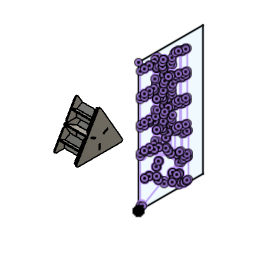
Table and Chair v10 (Autodesk Fusion 360 design; units mm, degrees)
Autodesk Fusion 360 part; units mm, degrees
note: some values were not read from the file. Chosen so that the rebuilt part matches the saved one: which bodies a step acts on.
(part 1 of 4)
sketch "Sketch1" plane through (0, 0, 0) normal (1, 0, 0) x (0, 1, 0)
  line L0 (0, 527.9291) -> (-457.2, -263.9645)
  line L1 (-457.2, -263.9645) -> (457.2, -263.9645)
  line L2 (457.2, -263.9645) -> (0, 527.9291)
  line L3 (0, 0) -> (0, 527.9291) construction
  line L4 (0, 0) -> (-228.6, 131.9823) construction
  line L5 (0, 0) -> (0, -263.9645) construction
  line L6 (0, 0) -> (228.6, 131.9823) construction
  line L7 (-228.6, 131.9823) -> (228.6, 131.9823)
  line L8 (-228.6, 131.9823) -> (0, -263.9645)
  line L9 (0, -263.9645) -> (228.6, 131.9823)
  line L10 (-114.3, -65.9911) -> (-228.6, -131.9823) construction
  line L11 (-228.6, -131.9823) -> (-342.9, -65.9911) construction
  line L12 (-228.6, -131.9823) -> (-228.6, -263.9645) construction
  line L13 (-118.8, -58.1969) -> (-228.6, -121.59)
  line L14 (-228.6, -121.59) -> (-338.4, -58.1969)
  line L15 (-109.8, -73.7854) -> (-219.6, -137.1784)
  line L16 (-219.6, -137.1784) -> (-219.6, -263.9645)
  line L17 (-237.6, -137.1784) -> (-347.4, -73.7854)
  line L18 (-237.6, -137.1784) -> (-237.6, -263.9645)
  line L19 (-228.6, -121.59) -> (-237.6, -137.1784)
  line L20 (-228.6, -121.59) -> (-219.6, -137.1784)
  line L21 (-219.6, -137.1784) -> (-237.6, -137.1784)
  line L22 (-228.6, 113.9823) -> (-441.6115, -254.9645)
  line L23 (-441.6115, -254.9645) -> (-15.5885, -254.9645)
  line L24 (-15.5885, -254.9645) -> (-228.6, 113.9823)
  line L25 (0, 10.3923) -> (-224.1, 139.7765)
  line L26 (0, 10.3923) -> (224.1, 139.7765)
  line L27 (-9, -5.1962) -> (-233.1, 124.188)
  line L28 (-9, -5.1962) -> (-9, -263.9645)
  line L29 (9, -5.1962) -> (9, -263.9645)
  line L30 (9, -5.1962) -> (233.1, 124.188)
  line L31 (-9, -5.1962) -> (9, -5.1962)
  line L32 (0, 10.3923) -> (9, -5.1962)
  line L33 (-9, -5.1962) -> (0, 10.3923)
  line L34 (0, 0, 0) -> (0, 0, 60) construction
  line L35 (-228.6, -131.9823, 0) -> (-228.6, -131.9823, 60) construction
  dimension "d693" = 3.05
  constraint coincident L3.start L4.start
  constraint equal L0 L1
  constraint equal L1 L2
  constraint vertical L3
  constraint midpoint L0 L4.end
  constraint midpoint L1 L5.end
  constraint midpoint L2 L6.end
  constraint equal L4 L6
  constraint equal L4 L5
  constraint midpoint L8 L10.start
  constraint perpendicular L8 L10
  constraint coincident L0 L11.end
  constraint coincident L1 L12.end
  constraint perpendicular L1 L12
  constraint perpendicular L0 L11
  constraint equal L10 L11
  constraint perpendicular L16 L23
  constraint parallel L8 L24
  constraint parallel L0 L22
  measures "d1" distance of L0.start L0.end
  measures "d6" distance of L0 L22
  measures "d7" distance of L1 L23
  measures "d8" distance of L8 L24
  measures "d35" distance of L3.start L4.start
  measures "d36" distance of L10.end L11.start
extrude "Extrude1" add sketch "Sketch1" along normal blind 18 makes body 1
extrude "Extrude2" add sketch "Sketch1" against normal blind 410 separate body contours L8 L9 L28 L29 L31 | L1 L9 L29 | L1 L8 L28 makes body 2
pattern_circular "C-Pattern1" count 3 over 360 about axis through (0, 0, 0) along (1, 0, 0) of bodies 2 makes body 3 at (-136.6667, 79.2, 35.3338) makes body 4 at (-273.3333, -70.2, 50.9223)
extrude "Extrude3" add sketch "Sketch1" against normal blind 18 from surface at -18 separate body contours L13 L14 L22 L24 | L14 L17 L19 L22 | L13 L15 L20 L24 | L17 L18 L22 L23 | L19 L20 L21 | L15 L16 L23 L24 | L16 L18 L21 L23 makes body 5
sketch "Sketch2" plane through (-410, 0, 0) normal (-1, 0, 0) x (0, -1, 0)
  line L0 (-224.1, 139.7765) -> (-233.1, 124.188)
  line L1 (-233.1, 124.188) -> (-9, -5.1962)
  line L2 (-9, -5.1962) -> (0, 10.3923)
  line L3 (0, 10.3923) -> (-224.1, 139.7765)
  line L4 (233.1, 124.188) -> (224.1, 139.7765)
  line L5 (224.1, 139.7765) -> (0, 10.3923)
  line L6 (0, 10.3923) -> (9, -5.1962)
  line L7 (9, -5.1962) -> (233.1, 124.188)
  line L8 (-9, -263.9645) -> (9, -263.9645)
  line L9 (9, -263.9645) -> (9, -5.1962)
  line L10 (9, -5.1962) -> (-9, -5.1962)
  line L11 (-9, -5.1962) -> (-9, -263.9645)
  line L12 (9, -134.5803) -> (-9, -134.5803) construction
  line L13 (9, -179.5803) -> (-9, -179.5803)
  line L14 (9, -89.5803) -> (-9, -89.5803)
  line L15 (-224.1, 139.7765) -> (224.1, 139.7765)
  line L16 (-233.1, 124.188) -> (-9, -263.9645)
  line L17 (233.1, 124.188) -> (9, -263.9645)
  line L18 (-4.5, 2.5981) -> (9, -5.1962) construction
  line L19 (0, -5.1962) -> (0, 10.3923) construction
  line L20 (73.0789, 52.5844) -> (82.0789, 36.9959)
  line L21 (151.0211, 97.5844) -> (160.0211, 81.9959)
  line L22 (-82.0789, 36.9959) -> (-73.0789, 52.5844)
  line L23 (-160.0211, 81.9959) -> (-151.0211, 97.5844)
  dimension "d34" = 90
  dimension "d38" = 360
  constraint midpoint L9 L12.start
  constraint midpoint L11 L12.end
  constraint coincident L9 L13.start
  constraint coincident L11 L13.end
  constraint perpendicular L11 L13
  constraint coincident L9 L14.start
  constraint coincident L11 L14.end
  constraint perpendicular L11 L14
  constraint symmetric L12 L13 L14
  constraint coincident L0.start L3.end
  constraint coincident L4.end L5.start
  constraint coincident L0.end L1.start
  constraint coincident L8.start L11.end
  constraint coincident L7 L4.start
  constraint coincident L8.end L9.start
  constraint coincident L4.start L7.end
  constraint midpoint L2 L18.start
  constraint coincident L6.end L7.start
  constraint midpoint L10 L19.start
  constraint coincident L2.end L3.start
  constraint coincident L19 origin
  constraint coincident L18 origin
  measures "d34" distance of L13 L14
extrude "Extrude5" add sketch "Sketch2" along normal blind 18 separate body contours L0 L1 L3 L23 | L3 L5 L15 | L1 L11 L16 | L4 L5 L7 L21 | L8 L9 L11 L13 | L1 L2 L3 L22 | L7 L9 L17 | L2 L6 L10 | L5 L6 L7 L20 | L9 L10 L11 L14 makes body 6
extrude "Extrude6" add sketch "Sketch2" along normal blind 18 contours L1 L3 L22 L23 | L5 L7 L20 L21 | L9 L11 L13 L14 bodies 2 3 4
ref_plane "WorkPlane2" through (-205, 0, -134.5803) normal (-1, 0, 0) x (0, 0, 1)
mirror "Mirror2" about plane through (-205, 0, -134.5803) normal (-1, 0, 0) of "Extrude6"
combine "Combine1" operation cut target body 1 tool bodies 3 2 4 keep tools
move_face "OffsetFaces1" offset -0.1 24 faces at (6, -3, -179.5803) (6, -3, -89.5803) (12, 99.0596, 67.5844) (12, 9, -119.5803) (12, -99.0596, 67.5844) (6, 108.0596, 51.9959) (6, -9, -119.5803) (12, -108.0596, 51.9959) (6, 157.0211, 87.1921) (6, -76.0789, 47.3883) (6, 79.0789, 42.1921) (6, -154.0211, 92.3883) (-416, 79.0789, 42.1921) (-416, 157.0211, 87.1921) (-416, 99.0596, 67.5844) (-422, 134.0404, 66.9959) (-416, -76.0789, 47.3883) (-416, -154.0211, 92.3883) (-416, 9, -119.5803) (-416, -125.0404, 82.5844) (-416, -3, -89.5803) (-416, -108.0596, 51.9959) (-416, -3, -179.5803) (-416, -9, -149.5803) on bodies 1 6
ref_plane "WorkPlane1" through (-223, 0, -62.094) normal (-1, 0, 0) x (0, 0, 1)
fillet "Fillet1" radius 30 6 edges at (9, -457.2, -263.9645) (9, 457.2, -263.9645) (9, 0, 527.9291) (-27, -441.6115, -254.9645) (-27, -15.5885, -254.9645) (-27, -228.6, 113.9823) on bodies 1 5
mirror "Mirror1" about plane through (-223, 0, -62.094) normal (-1, 0, 0) of bodies 5 makes body 7
extrude "Extrude4" add sketch "Sketch1" against normal up to surface (374 mm away) from surface at -36 separate body contours L16 L18 L21 L23 makes body 8
pattern_circular "C-Pattern2" count 3 over 360 about axis through (0, -228.6, -131.9823) along (1, 0, 0) of bodies 8 makes body 9 at (-285.3333, -185.5981, -117.5474) makes body 10 at (-160.6667, -262.6019, -101.9589)
sketch "Sketch3" plane through (-428, 0, 0) normal (-1, 0, 0) x (0, -1, 0)
  arc A0 (254.5808, 68.9823) -> (202.6192, 68.9823) centre (228.6, 53.9823) ccw
  line L0 (202.6192, 68.9823) -> (41.5692, -209.9645)
  arc A1 (41.5692, -209.9645) -> (67.55, -254.9645) centre (67.55, -224.9645) ccw
  line L1 (67.55, -254.9645) -> (389.65, -254.9645)
  arc A2 (389.65, -254.9645) -> (415.6308, -209.9645) centre (389.65, -224.9645) ccw
  line L2 (415.6308, -209.9645) -> (254.5808, 68.9823)
  line L3 (339.6058, -78.2854) -> (330.6058, -62.6969)
  line L4 (330.6058, -62.6969) -> (228.6, -121.59)
  line L5 (228.6, -121.59) -> (237.6, -137.1784)
  line L6 (237.6, -137.1784) -> (339.6058, -78.2854)
  line L7 (126.5942, -62.6969) -> (117.5942, -78.2854)
  line L8 (117.5942, -78.2854) -> (219.6, -137.1784)
  line L9 (219.6, -137.1784) -> (228.6, -121.59)
  line L10 (228.6, -121.59) -> (126.5942, -62.6969)
  line L11 (219.6, -254.9645) -> (237.6, -254.9645)
  line L12 (237.6, -254.9645) -> (237.6, -137.1784)
  line L13 (237.6, -137.1784) -> (219.6, -137.1784)
  line L14 (219.6, -137.1784) -> (219.6, -254.9645)
  line L15 (168.5971, -107.7319) -> (177.5971, -92.1434) construction
  line L16 (146.9465, -95.2319) -> (155.9465, -79.6434)
  line L17 (190.2477, -120.2319) -> (199.2477, -104.6434)
  line L18 (228.6, -121.59) -> (228.6, -137.1784)
  line L19 (224.1, -129.3842) -> (237.6, -137.1784)
  line L20 (237.6, -221.0715) -> (219.6, -221.0715)
  line L21 (237.6, -171.0715) -> (219.6, -171.0715)
  line L22 (301.2535, -79.6434) -> (310.2535, -95.2319)
  line L23 (257.9523, -104.6434) -> (266.9523, -120.2319)
  point P0 (228.6, -131.9823)
  dimension "d45" = 50
  dimension "d47" = 360
  constraint midpoint L8 L15.start
  constraint midpoint L10 L15.end
  constraint coincident L8 L16.start
  constraint coincident L10 L16.end
  constraint perpendicular L10 L16
  constraint coincident L8 L17.start
  constraint coincident L10 L17.end
  constraint perpendicular L10 L17
  constraint symmetric L15 L16 L17
  constraint coincident L4.end L5.start
  constraint midpoint L13 L18.end
  constraint midpoint L9 L19.start
  constraint coincident L5.end L6.start
  constraint coincident L19 P0
  constraint coincident L18 P0
  measures "d45" distance of L16 L17
extrude "Extrude7" add sketch "Sketch3" against normal up to surface (18 mm away) separate body contours L4 L6 L22 L23 | L8 L10 L16 L17 | L12 L14 L20 L21 makes body 11 at (-422, -281.386, -111.8986) makes body 12 at (-428, -181.814, -101.5063) makes body 13 at (-422, -219.6, -187.7382)
ref_plane "WorkPlane3" through (-223, -228.6, -70.4911) normal (-1, 0, 0) x (0, 0, 1)
mirror "Mirror3" about plane through (-223, -228.6, -70.4911) normal (-1, 0, 0) of bodies 13 12 11 makes body 14 at (-24, -281.386, -111.8986) makes body 15 at (-18, -181.814, -101.5063) makes body 16 at (-24, -219.6, -187.7382)
combine "Combine2" operation add target body 9 tool bodies 12 15
combine "Combine3" operation add target body 10 tool bodies 11 14
combine "Combine4" operation add target body 8 tool bodies 13 16
combine "Combine5" operation cut target body 5 tool bodies 8 9 10 keep tools
combine "Combine6" operation cut target body 7 tool bodies 10 8 9 keep tools
move_face "OffsetFaces2" offset -0.1 24 faces at (-416, -237.6, -187.7382) (-422, -175.814, -111.8986) (-416, -219.6, -187.7382) (-422, -286.8198, -87.9768) (-422, -193.2477, -115.0357) (-422, -231.6, -171.0715) (-422, -231.6, -221.0715) (-416, -281.386, -111.8986) (-422, -304.2535, -84.8396) (-422, -184.814, -96.3101) (-422, -260.9523, -109.8396) (-422, -149.9465, -90.0357) (-24, -231.6, -171.0715) (-24, -304.2535, -84.8396) (-24, -281.386, -111.8986) (-30, -184.814, -96.3101) (-24, -231.6, -221.0715) (-30, -219.6, -187.7382) (-24, -193.2477, -115.0357) (-30, -272.386, -96.3101) (-30, -237.6, -187.7382) (-30, -175.814, -111.8986) (-24, -260.9523, -109.8396) (-24, -149.9465, -90.0357) on bodies 5 7
pattern_circular "C-Pattern3" count 3 over 360 about axis through (661.68, 0.1832, -0.2415) along (-1, 0, 0) of bodies 7 5 8 9 10 makes body 17 at (-18, -77.6648, 228.6417) makes body 18 at (-18, 237.326, -47.2647) makes body 19 at (-428, -77.6648, 228.6417) makes body 20 at (-428, 237.326, -47.2647) makes body 21 at (-285.3333, -43.302, 299.4332) makes body 22 at (-160.6667, 281.4517, -112.4195) makes body 23 at (-285.3333, -8.516, 208.0051) makes body 24 at (-285.3333, 184.8797, -96.831) makes body 25 at (-285.3333, 67.7038, 292.178) makes body 26 at (-285.3333, 219.6657, -204.9258)
copy_body "Body->Comp1" bodies 1 removing the originals makes body 27 in component "Component"
copy_body "Body->Comp2" bodies 2 removing the originals makes body 28 in component "Component'"
copy_body "Body->Comp3" bodies 3 removing the originals makes body 29 in component "Component''"
copy_body "Body->Comp4" bodies 4 removing the originals makes body 30 in component "Component'''"
copy_body "Body->Comp5" bodies 5 removing the originals makes body 31 in component "Component''''"
copy_body "Body->Comp6" bodies 6 removing the originals makes body 32 in component "Component'''''"
copy_body "Body->Comp7" bodies 7 removing the originals makes body 33 in component "Component''''''"
copy_body "Body->Comp8" bodies 8 removing the originals makes body 34 in component "Component'''''''"
copy_body "Body->Comp9" bodies 9 removing the originals makes body 35 in component "Component''''''''"
copy_body "Body->Comp10" bodies 10 removing the originals makes body 36 in component "Component'''''''''"
copy_body "Body->Comp11" bodies 17 removing the originals makes body 37 in component "Component''''''''''"
copy_body "Body->Comp12" bodies 18 removing the originals makes body 38 in component "Component'''''''''''"
copy_body "Body->Comp13" bodies 19 removing the originals makes body 39 in component "Component''''''''''''"
copy_body "Body->Comp14" bodies 20 removing the originals makes body 40 in component "Component'''''''''''''"
copy_body "Body->Comp15" bodies 21 removing the originals makes body 41 in component "Component''''''''''''''"
copy_body "Body->Comp16" bodies 22 removing the originals makes body 42 in component "Component'''''''''''''''"
copy_body "Body->Comp17" bodies 23 removing the originals makes body 43 in component "Component''''''''''''''''"
copy_body "Body->Comp18" bodies 24 removing the originals makes body 44 in component "Component'''''''''''''''''"
copy_body "Body->Comp19" bodies 25 removing the originals makes body 45 in component "Component''''''''''''''''''"
copy_body "Body->Comp20" bodies 26 removing the originals makes body 46 in component "Component'''''''''''''''''''"
sketch "Sketch4" plane through (18, 0, 0) normal (1, 0, 0) x (0, 1, 0)
  arc A0 (25.9808, 482.9291) -> (-25.9808, 482.9291) centre (0, 467.9291) ccw
  line L0 (-25.9808, 482.9291) -> (-431.2192, -218.9645)
  arc A1 (-431.2192, -218.9645) -> (-405.2385, -263.9645) centre (-405.2385, -233.9645) ccw
  line L1 (-405.2385, -263.9645) -> (405.2385, -263.9645)
  arc A2 (405.2385, -263.9645) -> (431.2192, -218.9645) centre (405.2385, -233.9645) ccw
  line L2 (431.2192, -218.9645) -> (25.9808, 482.9291)
  line L3 (-72.9423, 52.621) -> (-82.0423, 36.8593)
  line L4 (-82.0423, 36.8593) -> (-160.1577, 81.9593)
  line L5 (-160.1577, 81.9593) -> (-151.0577, 97.721)
  line L6 (-151.0577, 97.721) -> (-72.9423, 52.621)
  line L7 (-9.1, -89.4803) -> (9.1, -89.4803)
  line L8 (9.1, -89.4803) -> (9.1, -179.6803)
  line L9 (9.1, -179.6803) -> (-9.1, -179.6803)
  line L10 (-9.1, -179.6803) -> (-9.1, -89.4803)
  line L11 (82.0423, 36.8593) -> (72.9423, 52.621)
  line L12 (72.9423, 52.621) -> (151.0577, 97.721)
  line L13 (151.0577, 97.721) -> (160.1577, 81.9593)
  line L14 (160.1577, 81.9593) -> (82.0423, 36.8593)
  line L15 (700, 919.2) -> (3138.4, 919.2)
  line L16 (3138.4, 919.2) -> (3138.4, -1519.2)
  line L17 (3138.4, -1519.2) -> (700, -1519.2)
  line L18 (700, -1519.2) -> (700, 919.2)
  dimension "d53" = 2438.4
  dimension "d54" = 2438.4
  constraint horizontal L15
  constraint vertical L16
  constraint horizontal L17
  constraint vertical L18
  measures "d53" distance of L15.start L15.end
  measures "d54" distance of L15.start L17.end
extrude "Extrude1'" add sketch "Sketch4" along normal blind 1 separate body contours L15 L16 L17 L18 makes body 47 in component "sheet"
other "Arrange1"
ref_plane "WorkPlane56" through (39, 1561.7871, -1471.2) normal (1, 0, 0) x (0, 0, 1)
sketch "Sketch58" plane through (39, 1561.7871, -1471.2) normal (1, 0, 0) x (0, 0, 1)
  line L0 (0, 0) -> (0, 33.8931) construction
  line L1 (-18, 0) -> (0, 0) construction
  line L2 (0, 0) -> (-2.1567, 2.1567) construction
  circle A0 centre (-2.1567, 2.1567) radius 3.05
  dimension "d525" = 3.05
  constraint coincident L0.start L1.end
  constraint coincident L0.start A0
  measures "d525" distance of L0.start L2.end
sweep "Sweep5" cut profiles "Sketch58" along 1 edges at (-410, -151.4465, -87.4377) section 1 sketch seen with x (0, -0.5, 0.866025) y (0, -0.866025, -0.5) z (1, 0, 0) at (1061.2, 1225.1008, 651.8867) on bodies 35 bodies 35 in component "Component''''''''"
ref_plane "WorkPlane57" through (57, 1611.7871, -1471.2) normal (-1, 0, 0) x (0, 0, -1)
sketch "Sketch59" plane through (57, 1611.7871, -1471.2) normal (-1, 0, 0) x (0, 0, -1)
  line L0 (0, 0) -> (0, -33.8931) construction
  line L1 (18, 0) -> (0, 0) construction
  line L2 (0, 0) -> (2.1567, -2.1567) construction
  circle A0 centre (2.1567, -2.1567) radius 3.05
  dimension "d533" = 3.05
  constraint coincident L0.start L1.end
  constraint coincident L0.start A0
  measures "d533" distance of L0.start L2.end
sweep "Sweep6" cut profiles "Sketch59" along 1 edges at (-410, -194.7477, -112.4377) section 1 sketch seen with x (0, -0.5, 0.866025) y (0, -0.866025, -0.5) z (1, 0, 0) at (1061.2, 1225.1008, 651.8867) on bodies 35 bodies 35 in component "Component''''''''"
ref_plane "WorkPlane58" through (57, 1561.7871, -1097.2) normal (-1, 0, 0) x (0, 0, -1)
sketch "Sketch60" plane through (57, 1561.7871, -1097.2) normal (-1, 0, 0) x (0, 0, -1)
  line L0 (0, 0) -> (0, 33.8931) construction
  line L1 (-18, 0) -> (0, 0) construction
  line L2 (0, 0) -> (-2.1567, 2.1567) construction
  circle A0 centre (-2.1567, 2.1567) radius 3.05
  dimension "d541" = 3.05
  constraint coincident L0.start L1.end
  constraint coincident L0.start A0
  measures "d541" distance of L0.start L2.end
sweep "Sweep7" cut profiles "Sketch60" along 1 edges at (-36, -151.4465, -87.4377) section 1 sketch seen with x (0, -0.5, 0.866025) y (0, -0.866025, -0.5) z (1, 0, 0) at (1061.2, 1225.1008, 651.8867) on bodies 35 bodies 35 in component "Component''''''''"
ref_plane "WorkPlane59" through (39, 1611.7871, -1097.2) normal (1, 0, 0) x (0, 0, 1)
sketch "Sketch61" plane through (39, 1611.7871, -1097.2) normal (1, 0, 0) x (0, 0, 1)
  line L0 (0, 0) -> (0, -33.8931) construction
  line L1 (18, 0) -> (0, 0) construction
  line L2 (0, 0) -> (2.1567, -2.1567) construction
  circle A0 centre (2.1567, -2.1567) radius 3.05
  dimension "d549" = 3.05
  constraint coincident L0.start L1.end
  constraint coincident L0.start A0
  measures "d549" distance of L0.start L2.end
sweep "Sweep8" cut profiles "Sketch61" along 1 edges at (-36, -194.7477, -112.4377) section 1 sketch seen with x (0, -0.5, 0.866025) y (0, -0.866025, -0.5) z (1, 0, 0) at (1061.2, 1225.1008, 651.8867) on bodies 35 bodies 35 in component "Component''''''''"
ref_plane "WorkPlane60" through (57, 1611.7872, -1041.2) normal (-1, 0, 0) x (0, 0, -1)
sketch "Sketch62" plane through (57, 1611.7872, -1041.2) normal (-1, 0, 0) x (0, 0, -1)
  line L0 (0, 0) -> (0, -33.8931) construction
  line L1 (18, 0) -> (0, 0) construction
  line L2 (0, 0) -> (2.1567, -2.1567) construction
  circle A0 centre (2.1567, -2.1567) radius 3.05
  dimension "d557" = 3.05
  constraint coincident L0.start L1.end
  constraint coincident L0.start A0
  measures "d557" distance of L0.start L2.end
sweep "Sweep5'" cut profiles "Sketch62" along 1 edges at (-36, -262.4523, -112.4377) section 1 sketch seen with x (0, 0.5, 0.866025) y (0, 0.866025, -0.5) z (-1, 0, 0) at (-1077.2, -1682.3009, 651.8867) on bodies 36 bodies 36 in component "Component'''''''''"
ref_plane "WorkPlane61" through (39, 1561.7872, -1041.2) normal (1, 0, 0) x (0, 0, 1)
sketch "Sketch63" plane through (39, 1561.7872, -1041.2) normal (1, 0, 0) x (0, 0, 1)
  line L0 (0, 0) -> (0, 33.8931) construction
  line L1 (-18, 0) -> (0, 0) construction
  line L2 (0, 0) -> (-2.1567, 2.1567) construction
  circle A0 centre (-2.1567, 2.1567) radius 3.05
  dimension "d565" = 3.05
  constraint coincident L0.start L1.end
  constraint coincident L0.start A0
  measures "d565" distance of L0.start L2.end
sweep "Sweep6'" cut profiles "Sketch63" along 1 edges at (-36, -305.7535, -87.4377) section 1 sketch seen with x (0, 0.5, 0.866025) y (0, 0.866025, -0.5) z (-1, 0, 0) at (-1077.2, -1682.3009, 651.8867) on bodies 36 bodies 36 in component "Component'''''''''"
ref_plane "WorkPlane62" through (39, 1424.0012, -937.046) normal (1, 0, 0) x (0, 0, 1)
sketch "Sketch64" plane through (39, 1424.0012, -937.046) normal (1, 0, 0) x (0, 0, 1)
  line L0 (0, 0) -> (0, 33.8931) construction
  line L1 (-18, 0) -> (0, 0) construction
  line L2 (0, 0) -> (-2.1567, 2.1567) construction
  circle A0 centre (-2.1567, 2.1567) radius 3.05
  dimension "d573" = 3.05
  constraint coincident L0.start L1.end
  constraint coincident L0.start A0
  measures "d573" distance of L0.start L2.end
sweep "Sweep5''" cut profiles "Sketch64" along 1 edges at (-410, 305.8192, -87.9586) section 1 sketch seen with x (0, -0.5, 0.866025) y (0, -0.866025, -0.5) z (1, 0, 0) at (527.046, 1563.0405, 582.4728) on bodies 42 bodies 42 in component "Component'''''''''''''''"
ref_plane "WorkPlane63" through (57, 1474.0012, -937.046) normal (-1, 0, 0) x (0, 0, -1)
sketch "Sketch65" plane through (57, 1474.0012, -937.046) normal (-1, 0, 0) x (0, 0, -1)
  line L0 (0, 0) -> (0, -33.8931) construction
  line L1 (18, 0) -> (0, 0) construction
  line L2 (0, 0) -> (2.1567, -2.1567) construction
  circle A0 centre (2.1567, -2.1567) radius 3.05
  dimension "d581" = 3.05
  constraint coincident L0.start L1.end
  constraint coincident L0.start A0
  measures "d581" distance of L0.start L2.end
sweep "Sweep6''" cut profiles "Sketch65" along 1 edges at (-410, 262.518, -112.9586) section 1 sketch seen with x (0, -0.5, 0.866025) y (0, -0.866025, -0.5) z (1, 0, 0) at (527.046, 1563.0405, 582.4728) on bodies 42 bodies 42 in component "Component'''''''''''''''"
ref_plane "WorkPlane64" through (57, 1561.7872, -667.2) normal (-1, 0, 0) x (0, 0, -1)
sketch "Sketch66" plane through (57, 1561.7872, -667.2) normal (-1, 0, 0) x (0, 0, -1)
  line L0 (0, 0) -> (0, 33.8931) construction
  line L1 (-18, 0) -> (0, 0) construction
  line L2 (0, 0) -> (-2.1567, 2.1567) construction
  circle A0 centre (-2.1567, 2.1567) radius 3.05
  dimension "d589" = 3.05
  constraint coincident L0.start L1.end
  constraint coincident L0.start A0
  measures "d589" distance of L0.start L2.end
sweep "Sweep7'" cut profiles "Sketch66" along 1 edges at (-410, -305.7535, -87.4377) section 1 sketch seen with x (0, 0.5, 0.866025) y (0, 0.866025, -0.5) z (-1, 0, 0) at (-1077.2, -1682.3009, 651.8867) on bodies 36 bodies 36 in component "Component'''''''''"
ref_plane "WorkPlane65" through (39, 1611.7872, -667.2) normal (1, 0, 0) x (0, 0, 1)
sketch "Sketch67" plane through (39, 1611.7872, -667.2) normal (1, 0, 0) x (0, 0, 1)
  line L0 (0, 0) -> (0, -33.8931) construction
  line L1 (18, 0) -> (0, 0) construction
  line L2 (0, 0) -> (2.1567, -2.1567) construction
  circle A0 centre (2.1567, -2.1567) radius 3.05
  dimension "d597" = 3.05
  constraint coincident L0.start L1.end
  constraint coincident L0.start A0
  measures "d597" distance of L0.start L2.end
sweep "Sweep8'" cut profiles "Sketch67" along 1 edges at (-410, -262.4523, -112.4377) section 1 sketch seen with x (0, 0.5, 0.866025) y (0, 0.866025, -0.5) z (-1, 0, 0) at (-1077.2, -1682.3009, 651.8867) on bodies 36 bodies 36 in component "Component'''''''''"
ref_plane "WorkPlane66" through (39, 1474.0012, -563.046) normal (1, 0, 0) x (0, 0, 1)
sketch "Sketch68" plane through (39, 1474.0012, -563.046) normal (1, 0, 0) x (0, 0, 1)
  line L0 (0, 0) -> (0, -33.8931) construction
  line L1 (18, 0) -> (0, 0) construction
  line L2 (0, 0) -> (2.1567, -2.1567) construction
  circle A0 centre (2.1567, -2.1567) radius 3.05
  dimension "d605" = 3.05
  constraint coincident L0.start L1.end
  constraint coincident L0.start A0
  measures "d605" distance of L0.start L2.end
sweep "Sweep7''" cut profiles "Sketch68" along 1 edges at (-36, 262.518, -112.9586) section 1 sketch seen with x (0, -0.5, 0.866025) y (0, -0.866025, -0.5) z (1, 0, 0) at (527.046, 1563.0405, 582.4728) on bodies 42 bodies 42 in component "Component'''''''''''''''"
ref_plane "WorkPlane67" through (57, 1424.0012, -563.046) normal (-1, 0, 0) x (0, 0, -1)
sketch "Sketch69" plane through (57, 1424.0012, -563.046) normal (-1, 0, 0) x (0, 0, -1)
  line L0 (0, 0) -> (0, 33.8931) construction
  line L1 (-18, 0) -> (0, 0) construction
  line L2 (0, 0) -> (-2.1567, 2.1567) construction
  circle A0 centre (-2.1567, 2.1567) radius 3.05
  dimension "d613" = 3.05
  constraint coincident L0.start L1.end
  constraint coincident L0.start A0
  measures "d613" distance of L0.start L2.end
sweep "Sweep8''" cut profiles "Sketch69" along 1 edges at (-36, 305.8192, -87.9586) section 1 sketch seen with x (0, -0.5, 0.866025) y (0, -0.866025, -0.5) z (1, 0, 0) at (527.046, 1563.0405, 582.4728) on bodies 42 bodies 42 in component "Component'''''''''''''''"
ref_plane "WorkPlane68" through (57, 1589.3944, -543.0459) normal (-1, 0, 0) x (0, 0, -1)
sketch "Sketch70" plane through (57, 1589.3944, -543.0459) normal (-1, 0, 0) x (0, 0, -1)
  line L0 (0, 0) -> (0, -33.8931) construction
  line L1 (18, 0) -> (0, 0) construction
  line L2 (0, 0) -> (2.1567, -2.1567) construction
  circle A0 centre (2.1567, -2.1567) radius 3.05
  dimension "d621" = 3.05
  constraint coincident L0.start L1.end
  constraint coincident L0.start A0
  measures "d621" distance of L0.start L2.end
sweep "Sweep5'''" cut profiles "Sketch70" along 1 edges at (-36, -33.3682, 283.3056) section 1 sketch seen with x (0, 0.5, 0.866025) y (0, 0.866025, -0.5) z (-1, 0, 0) at (-579.0459, -1433.8242, 1036.4336) on bodies 41 bodies 41 in component "Component''''''''''''''"
ref_plane "WorkPlane69" through (39, 1539.3944, -543.0459) normal (1, 0, 0) x (0, 0, 1)
sketch "Sketch71" plane through (39, 1539.3944, -543.0459) normal (1, 0, 0) x (0, 0, 1)
  line L0 (0, 0) -> (0, 33.8931) construction
  line L1 (-18, 0) -> (0, 0) construction
  line L2 (0, 0) -> (-2.1567, 2.1567) construction
  circle A0 centre (-2.1567, 2.1567) radius 3.05
  dimension "d629" = 3.05
  constraint coincident L0.start L1.end
  constraint coincident L0.start A0
  measures "d629" distance of L0.start L2.end
sweep "Sweep6'''" cut profiles "Sketch71" along 1 edges at (-36, -76.6695, 308.3056) section 1 sketch seen with x (0, 0.5, 0.866025) y (0, 0.866025, -0.5) z (-1, 0, 0) at (-579.0459, -1433.8242, 1036.4336) on bodies 41 bodies 41 in component "Component''''''''''''''"
ref_plane "WorkPlane70" through (39, 1401.6083, -507.0458) normal (1, 0, 0) x (0, 0, 1)
sketch "Sketch72" plane through (39, 1401.6083, -507.0458) normal (1, 0, 0) x (0, 0, 1)
  line L0 (-18, 0) -> (0, 0) construction
  line L1 (0, 33.8931) -> (0, 0) construction
  line L2 (0, 0) -> (-2.1567, 2.1567) construction
  circle A0 centre (-2.1567, 2.1567) radius 3.05
  dimension "d637" = 3.05
  constraint coincident L0.end L1.end
  constraint coincident L0.end A0
  measures "d637" distance of L0.end L2.end
sweep "Sweep5''''" cut profiles "Sketch72" along 1 edges at (-36, 151.5122, -87.9586) section 1 sketch seen with x (0, 0.5, 0.866025) y (0, 0.866025, -0.5) z (-1, 0, 0) at (-543.0458, -1086.3162, 571.2763) on bodies 44 bodies 44 in component "Component'''''''''''''''''"
ref_plane "WorkPlane71" through (57, 1451.6083, -507.0458) normal (-1, 0, 0) x (0, 0, -1)
sketch "Sketch73" plane through (57, 1451.6083, -507.0458) normal (-1, 0, 0) x (0, 0, -1)
  line L0 (0, 0) -> (0, -33.8931) construction
  line L1 (18, 0) -> (0, 0) construction
  line L2 (0, 0) -> (2.1567, -2.1567) construction
  circle A0 centre (2.1567, -2.1567) radius 3.05
  dimension "d645" = 3.05
  constraint coincident L0.start L1.end
  constraint coincident L0.start A0
  measures "d645" distance of L0.start L2.end
sweep "Sweep6''''" cut profiles "Sketch73" along 1 edges at (-36, 194.8135, -112.9586) section 1 sketch seen with x (0, 0.5, 0.866025) y (0, 0.866025, -0.5) z (-1, 0, 0) at (-543.0458, -1086.3162, 571.2763) on bodies 44 bodies 44 in component "Component'''''''''''''''''"
ref_plane "WorkPlane72" through (57, 1539.3944, -169.0459) normal (-1, 0, 0) x (0, 0, -1)
sketch "Sketch74" plane through (57, 1539.3944, -169.0459) normal (-1, 0, 0) x (0, 0, -1)
  line L0 (0, 0) -> (0, 33.8931) construction
  line L1 (-18, 0) -> (0, 0) construction
  line L2 (0, 0) -> (-2.1567, 2.1567) construction
  circle A0 centre (-2.1567, 2.1567) radius 3.05
  dimension "d653" = 3.05
  constraint coincident L0.start L1.end
  constraint coincident L0.start A0
  measures "d653" distance of L0.start L2.end
sweep "Sweep7'''" cut profiles "Sketch74" along 1 edges at (-410, -76.6695, 308.3056) section 1 sketch seen with x (0, 0.5, 0.866025) y (0, 0.866025, -0.5) z (-1, 0, 0) at (-579.0459, -1433.8242, 1036.4336) on bodies 41 bodies 41 in component "Component''''''''''''''"
ref_plane "WorkPlane73" through (39, 1589.3944, -169.0459) normal (1, 0, 0) x (0, 0, 1)
sketch "Sketch75" plane through (39, 1589.3944, -169.0459) normal (1, 0, 0) x (0, 0, 1)
  line L0 (0, 0) -> (0, -33.8931) construction
  line L1 (18, 0) -> (0, 0) construction
  line L2 (0, 0) -> (2.1567, -2.1567) construction
  circle A0 centre (2.1567, -2.1567) radius 3.05
  dimension "d661" = 3.05
  constraint coincident L0.start L1.end
  constraint coincident L0.start A0
  measures "d661" distance of L0.start L2.end
sweep "Sweep8'''" cut profiles "Sketch75" along 1 edges at (-410, -33.3682, 283.3056) section 1 sketch seen with x (0, 0.5, 0.866025) y (0, 0.866025, -0.5) z (-1, 0, 0) at (-579.0459, -1433.8242, 1036.4336) on bodies 41 bodies 41 in component "Component''''''''''''''"
ref_plane "WorkPlane74" through (57, 1401.6083, -133.0458) normal (-1, 0, 0) x (0, 0, -1)
sketch "Sketch76" plane through (57, 1401.6083, -133.0458) normal (-1, 0, 0) x (0, 0, -1)
  line L0 (0, 0) -> (0, 33.8931) construction
  line L1 (-18, 0) -> (0, 0) construction
  line L2 (0, 0) -> (-2.1567, 2.1567) construction
  circle A0 centre (-2.1567, 2.1567) radius 3.05
  dimension "d669" = 3.05
  constraint coincident L0.start L1.end
  constraint coincident L0.start A0
  measures "d669" distance of L0.start L2.end
sweep "Sweep7''''" cut profiles "Sketch76" along 1 edges at (-410, 151.5122, -87.9586) section 1 sketch seen with x (0, 0.5, 0.866025) y (0, 0.866025, -0.5) z (-1, 0, 0) at (-543.0458, -1086.3162, 571.2763) on bodies 44 bodies 44 in component "Component'''''''''''''''''"
ref_plane "WorkPlane75" through (39, 1451.6083, -133.0458) normal (1, 0, 0) x (0, 0, 1)
sketch "Sketch77" plane through (39, 1451.6083, -133.0458) normal (1, 0, 0) x (0, 0, 1)
  line L0 (0, 0) -> (0, -33.8931) construction
  line L1 (18, 0) -> (0, 0) construction
  line L2 (0, 0) -> (2.1567, -2.1567) construction
  circle A0 centre (2.1567, -2.1567) radius 3.05
  dimension "d677" = 3.05
  constraint coincident L0.start L1.end
  constraint coincident L0.start A0
  measures "d677" distance of L0.start L2.end
sweep "Sweep8''''" cut profiles "Sketch77" along 1 edges at (-410, 194.8135, -112.9586) section 1 sketch seen with x (0, 0.5, 0.866025) y (0, 0.866025, -0.5) z (-1, 0, 0) at (-543.0458, -1086.3162, 571.2763) on bodies 44 bodies 44 in component "Component'''''''''''''''''"
ref_plane "WorkPlane76" through (39, 1539.3944, -113.0459) normal (1, 0, 0) x (0, 0, -1)
sketch "Sketch78" plane through (39, 1539.3944, -113.0459) normal (1, 0, 0) x (0, 0, -1)
  line L0 (18, 0) -> (0, 0) construction
  line L1 (0, -33.8931) -> (0, 0) construction
  line L2 (0, 0) -> (2.1567, -2.1567) construction
  circle A0 centre (2.1567, -2.1567) radius 3.05
  dimension "d685" = 3.05
  constraint coincident L0.end L1.end
  constraint coincident L0.end A0
  measures "d685" distance of L0.end L2.end
sweep "Sweep5'''''" cut profiles "Sketch78" along 1 edges at (-36, 0.484, 174.6718) section 1 sketch seen with x (0, -1, 0) y (0, 0, 1) z (-1, 0, 0) at (-149.0459, 48.484, -1364.7226) on bodies 43 bodies 43 in component "Component''''''''''''''''"
ref_plane "WorkPlane77" through (57, 1589.3944, -113.0459) normal (-1, 0, 0) x (0, 0, 1)
sketch "sketch 45411" plane through (57, 1589.3944, -113.0459) normal (-1, 0, 0) x (0, 0, 1)
  line L0 (0, 0) -> (0, 33.8931) construction
  line L1 (-18, 0) -> (0, 0) construction
  line L2 (0, 0) -> (-2.1567, 2.1567) construction
  circle A0 centre (-2.1567, 2.1567) radius 3.05
  constraint coincident L0.start L1.end
  constraint coincident L0.start A0
  measures "d693" distance of L0.start L2.end
sweep "Sweep6'''''" cut profiles "sketch 45411" along 1 edges at (-36, 0.484, 224.6718) section 1 sketch seen with x (0, -1, 0) y (0, 0, 1) z (-1, 0, 0) at (-149.0459, 48.484, -1364.7226) on bodies 43 bodies 43 in component "Component''''''''''''''''"
ref_plane "WorkPlane78" through (39, 1401.6084, -77.0459) normal (1, 0, 0) x (0, 0, -1)
sketch "Sketch80" plane through (39, 1401.6084, -77.0459) normal (1, 0, 0) x (0, 0, -1)
  line L0 (0, 0) -> (0, -33.8931) construction
  line L1 (18, 0) -> (0, 0) construction
  line L2 (0, 0) -> (2.1567, -2.1567) construction
  circle A0 centre (2.1567, -2.1567) radius 3.05
  dimension "d701" = 3.05
  constraint coincident L0.start L1.end
  constraint coincident L0.start A0
  measures "d701" distance of L0.start L2.end
sweep "Sweep5''''''" cut profiles "Sketch80" along 1 edges at (-36, 228.6657, -221.5924) section 1 sketch seen with x (0, -1, 0) y (0, 0, 1) z (-1, 0, 0) at (-113.0459, 276.6657, -1623.2008) on bodies 46 bodies 46 in component "Component'''''''''''''''''''"
ref_plane "WorkPlane79" through (57, 1451.6084, -77.0459) normal (-1, 0, 0) x (0, 0, 1)
sketch "Sketch81" plane through (57, 1451.6084, -77.0459) normal (-1, 0, 0) x (0, 0, 1)
  line L0 (0, 0) -> (0, 33.8931) construction
  line L1 (-18, 0) -> (0, 0) construction
  line L2 (0, 0) -> (-2.1567, 2.1567) construction
  circle A0 centre (-2.1567, 2.1567) radius 3.05
  dimension "d709" = 3.05
  constraint coincident L0.start L1.end
  constraint coincident L0.start A0
  measures "d709" distance of L0.start L2.end
sweep "Sweep6''''''" cut profiles "Sketch81" along 1 edges at (-36, 228.6657, -171.5924) section 1 sketch seen with x (0, -1, 0) y (0, 0, 1) z (-1, 0, 0) at (-113.0459, 276.6657, -1623.2008) on bodies 46 bodies 46 in component "Component'''''''''''''''''''"
ref_plane "WorkPlane80" through (57, 1539.3944, 260.9541) normal (-1, 0, 0) x (0, 0, 1)
sketch "Sketch82" plane through (57, 1539.3944, 260.9541) normal (-1, 0, 0) x (0, 0, 1)
  line L0 (0, 0) -> (0, -33.8931) construction
  line L1 (18, 0) -> (0, 0) construction
  line L2 (0, 0) -> (2.1567, -2.1567) construction
  circle A0 centre (2.1567, -2.1567) radius 3.05
  dimension "d717" = 3.05
  constraint coincident L0.start L1.end
  constraint coincident L0.start A0
  measures "d717" distance of L0.start L2.end
sweep "Sweep7'''''" cut profiles "Sketch82" along 1 edges at (-410, 0.484, 174.6718) section 1 sketch seen with x (0, -1, 0) y (0, 0, 1) z (-1, 0, 0) at (-149.0459, 48.484, -1364.7226) on bodies 43 bodies 43 in component "Component''''''''''''''''"
ref_plane "WorkPlane81" through (39, 1589.3944, 260.9541) normal (1, 0, 0) x (0, 0, -1)
sketch "Sketch83" plane through (39, 1589.3944, 260.9541) normal (1, 0, 0) x (0, 0, -1)
  line L0 (0, 0) -> (0, 33.8931) construction
  line L1 (-18, 0) -> (0, 0) construction
  line L2 (0, 0) -> (-2.1567, 2.1567) construction
  circle A0 centre (-2.1567, 2.1567) radius 3.05
  dimension "d725" = 3.05
  constraint coincident L0.start L1.end
  constraint coincident L0.start A0
  measures "d725" distance of L0.start L2.end
sweep "Sweep8'''''" cut profiles "Sketch83" along 1 edges at (-410, 0.484, 224.6718) section 1 sketch seen with x (0, -1, 0) y (0, 0, 1) z (-1, 0, 0) at (-149.0459, 48.484, -1364.7226) on bodies 43 bodies 43 in component "Component''''''''''''''''"
ref_plane "WorkPlane82" through (57, 1401.6084, 296.9541) normal (-1, 0, 0) x (0, 0, 1)
sketch "Sketch84" plane through (57, 1401.6084, 296.9541) normal (-1, 0, 0) x (0, 0, 1)
  line L0 (0, 0) -> (0, -33.8931) construction
  line L1 (18, 0) -> (0, 0) construction
  line L2 (0, 0) -> (2.1567, -2.1567) construction
  circle A0 centre (2.1567, -2.1567) radius 3.05
  dimension "d733" = 3.05
  constraint coincident L0.start L1.end
  constraint coincident L0.start A0
  measures "d733" distance of L0.start L2.end
sweep "Sweep7''''''" cut profiles "Sketch84" along 1 edges at (-410, 228.6657, -221.5924) section 1 sketch seen with x (0, -1, 0) y (0, 0, 1) z (-1, 0, 0) at (-113.0459, 276.6657, -1623.2008) on bodies 46 bodies 46 in component "Component'''''''''''''''''''"
ref_plane "WorkPlane83" through (39, 1451.6084, 296.9541) normal (1, 0, 0) x (0, 0, -1)
sketch "Sketch85" plane through (39, 1451.6084, 296.9541) normal (1, 0, 0) x (0, 0, -1)
  line L0 (0, 0) -> (0, 33.8931) construction
  line L1 (-18, 0) -> (0, 0) construction
  line L2 (0, 0) -> (-2.1567, 2.1567) construction
  circle A0 centre (-2.1567, 2.1567) radius 3.05
  dimension "d741" = 3.05
  constraint coincident L0.start L1.end
  constraint coincident L0.start A0
  measures "d741" distance of L0.start L2.end
sweep "Sweep8''''''" cut profiles "Sketch85" along 1 edges at (-410, 228.6657, -171.5924) section 1 sketch seen with x (0, -1, 0) y (0, 0, 1) z (-1, 0, 0) at (-113.0459, 276.6657, -1623.2008) on bodies 46 bodies 46 in component "Component'''''''''''''''''''"
ref_plane "WorkPlane84" through (57, 1589.3945, 316.9541) normal (-1, 0, 0) x (0, 0, 1)
sketch "Sketch86" plane through (57, 1589.3945, 316.9541) normal (-1, 0, 0) x (0, 0, 1)
  line L0 (0, 0) -> (0, 33.8931) construction
  line L1 (-18, 0) -> (0, 0) construction
  line L2 (0, 0) -> (-2.1567, 2.1567) construction
  circle A0 centre (-2.1567, 2.1567) radius 3.05
  dimension "d749" = 3.05
  constraint coincident L0.start L1.end
  constraint coincident L0.start A0
  measures "d749" distance of L0.start L2.end
sweep "Sweep5'''''''" cut profiles "Sketch86" along 1 edges at (-36, 77.6375, 308.3056) section 1 sketch seen with x (0, -0.5, 0.866025) y (0, 0.866025, 0.5) z (-1, 0, 0) at (280.9541, -1274.8185, -527.9609) on bodies 45 bodies 45 in component "Component''''''''''''''''''"
ref_plane "WorkPlane85" through (39, 1539.3945, 316.9541) normal (1, 0, 0) x (0, 0, -1)
sketch "Sketch87" plane through (39, 1539.3945, 316.9541) normal (1, 0, 0) x (0, 0, -1)
  line L0 (0, 0) -> (0, -33.8931) construction
  line L1 (18, 0) -> (0, 0) construction
  line L2 (0, 0) -> (2.1567, -2.1567) construction
  circle A0 centre (2.1567, -2.1567) radius 3.05
  dimension "d757" = 3.05
  constraint coincident L0.start L1.end
  constraint coincident L0.start A0
  measures "d757" distance of L0.start L2.end
sweep "Sweep6'''''''" cut profiles "Sketch87" along 1 edges at (-36, 34.3363, 283.3056) section 1 sketch seen with x (0, -0.5, 0.866025) y (0, 0.866025, 0.5) z (-1, 0, 0) at (280.9541, -1274.8185, -527.9609) on bodies 45 bodies 45 in component "Component''''''''''''''''''"
ref_plane "WorkPlane86" through (57, 1451.6084, 352.9541) normal (-1, 0, 0) x (0, 0, 1)
sketch "Sketch88" plane through (57, 1451.6084, 352.9541) normal (-1, 0, 0) x (0, 0, 1)
  line L0 (0, 0) -> (0, 33.8931) construction
  line L1 (-18, 0) -> (0, 0) construction
  line L2 (0, 0) -> (-2.1567, 2.1567) construction
  circle A0 centre (-2.1567, 2.1567) radius 3.05
  dimension "d765" = 3.05
  constraint coincident L0.start L1.end
  constraint coincident L0.start A0
  measures "d765" distance of L0.start L2.end
sweep "Sweep5''''''''" cut profiles "Sketch88" along 1 edges at (-36, -228.6, -171.0715) section 1 sketch seen with x (0, -1, 0) y (0, 0, 1) z (-1, 0, 0) at (316.9541, -180.6, -1622.6799) on bodies 34 bodies 34 in component "Component'''''''"
ref_plane "WorkPlane87" through (39, 1401.6084, 352.9541) normal (1, 0, 0) x (0, 0, -1)
sketch "Sketch89" plane through (39, 1401.6084, 352.9541) normal (1, 0, 0) x (0, 0, -1)
  line L0 (0, 0) -> (0, -33.8931) construction
  line L1 (18, 0) -> (0, 0) construction
  line L2 (0, 0) -> (2.1567, -2.1567) construction
  circle A0 centre (2.1567, -2.1567) radius 3.05
  dimension "d773" = 3.05
  constraint coincident L0.start L1.end
  constraint coincident L0.start A0
  measures "d773" distance of L0.start L2.end
sweep "Sweep6''''''''" cut profiles "Sketch89" along 1 edges at (-36, -228.6, -221.0715) section 1 sketch seen with x (0, -1, 0) y (0, 0, 1) z (-1, 0, 0) at (316.9541, -180.6, -1622.6799) on bodies 34 bodies 34 in component "Component'''''''"
ref_plane "WorkPlane88" through (57, 1539.3945, 690.9541) normal (-1, 0, 0) x (0, 0, 1)
sketch "Sketch90" plane through (57, 1539.3945, 690.9541) normal (-1, 0, 0) x (0, 0, 1)
  line L0 (0, 0) -> (0, -33.8931) construction
  line L1 (18, 0) -> (0, 0) construction
  line L2 (0, 0) -> (2.1567, -2.1567) construction
  circle A0 centre (2.1567, -2.1567) radius 3.05
  dimension "d781" = 3.05
  constraint coincident L0.start L1.end
  constraint coincident L0.start A0
  measures "d781" distance of L0.start L2.end
sweep "Sweep7'''''''" cut profiles "Sketch90" along 1 edges at (-410, 34.3363, 283.3056) section 1 sketch seen with x (0, -0.5, 0.866025) y (0, 0.866025, 0.5) z (-1, 0, 0) at (280.9541, -1274.8185, -527.9609) on bodies 45 bodies 45 in component "Component''''''''''''''''''"
ref_plane "WorkPlane89" through (39, 1589.3945, 690.9541) normal (1, 0, 0) x (0, 0, -1)
sketch "Sketch91" plane through (39, 1589.3945, 690.9541) normal (1, 0, 0) x (0, 0, -1)
  line L0 (0, 0) -> (0, 33.8931) construction
  line L1 (-18, 0) -> (0, 0) construction
  line L2 (0, 0) -> (-2.1567, 2.1567) construction
  circle A0 centre (-2.1567, 2.1567) radius 3.05
  dimension "d789" = 3.05
  constraint coincident L0.start L1.end
  constraint coincident L0.start A0
  measures "d789" distance of L0.start L2.end
sweep "Sweep8'''''''" cut profiles "Sketch91" along 1 edges at (-410, 77.6375, 308.3056) section 1 sketch seen with x (0, -0.5, 0.866025) y (0, 0.866025, 0.5) z (-1, 0, 0) at (280.9541, -1274.8185, -527.9609) on bodies 45 bodies 45 in component "Component''''''''''''''''''"
ref_plane "WorkPlane90" through (57, 1401.6084, 726.9541) normal (-1, 0, 0) x (0, 0, 1)
sketch "Sketch92" plane through (57, 1401.6084, 726.9541) normal (-1, 0, 0) x (0, 0, 1)
  line L0 (0, 0) -> (0, -33.8931) construction
  line L1 (18, 0) -> (0, 0) construction
  line L2 (0, 0) -> (2.1567, -2.1567) construction
  circle A0 centre (2.1567, -2.1567) radius 3.05
  dimension "d797" = 3.05
  constraint coincident L0.start L1.end
  constraint coincident L0.start A0
  measures "d797" distance of L0.start L2.end
sweep "Sweep7''''''''" cut profiles "Sketch92" along 1 edges at (-410, -228.6, -221.0715) section 1 sketch seen with x (0, -1, 0) y (0, 0, 1) z (-1, 0, 0) at (316.9541, -180.6, -1622.6799) on bodies 34 bodies 34 in component "Component'''''''"
ref_plane "WorkPlane91" through (39, 1451.6084, 726.9541) normal (1, 0, 0) x (0, 0, -1)
sketch "Sketch93" plane through (39, 1451.6084, 726.9541) normal (1, 0, 0) x (0, 0, -1)
  line L0 (0, 0) -> (0, 33.8931) construction
  line L1 (-18, 0) -> (0, 0) construction
  line L2 (0, 0) -> (-2.1567, 2.1567) construction
  circle A0 centre (-2.1567, 2.1567) radius 3.05
  dimension "d805" = 3.05
  constraint coincident L0.start L1.end
  constraint coincident L0.start A0
  measures "d805" distance of L0.start L2.end
sweep "Sweep8''''''''" cut profiles "Sketch93" along 1 edges at (-410, -228.6, -171.0715) section 1 sketch seen with x (0, -1, 0) y (0, 0, 1) z (-1, 0, 0) at (316.9541, -180.6, -1622.6799) on bodies 34 bodies 34 in component "Component'''''''"
ref_plane "WorkPlane92" through (57, 814.3842, 757.2001) normal (-1, 0, 0) x (0, 0, -1)
sketch "Sketch94" plane through (57, 814.3842, 757.2001) normal (-1, 0, 0) x (0, 0, -1)
  line L0 (0, 0) -> (0, 84.3842) construction
  line L1 (0, 0) -> (-18, 0) construction
  line L2 (0, 0) -> (-2.1567, 2.1567) construction
  circle A0 centre (-2.1567, 2.1567) radius 3.05
  dimension "d813" = 3.05
  constraint coincident L0.start L1.start
  constraint coincident L0.start A0
  measures "d813" distance of L0.start L2.end
sweep "Sweep5'''''''''" cut profiles "Sketch94" along 1 edges at (-410, -155.5211, 89.7902) section 1 sketch seen with x (0, 0.5, 0.866025) y (0, 0.866025, -0.5) z (-1, 0, 0) at (347.2001, -884.7986, 455.4131) on bodies 30 bodies 30 in component "Component'''"
ref_plane "WorkPlane93" through (39, 904.3842, 757.2001) normal (1, 0, 0) x (0, 0, 1)
sketch "Sketch95" plane through (39, 904.3842, 757.2001) normal (1, 0, 0) x (0, 0, 1)
  line L0 (0, 0) -> (0, -84.3842) construction
  line L1 (0, 0) -> (18, 0) construction
  line L2 (0, 0) -> (2.1567, -2.1567) construction
  circle A0 centre (2.1567, -2.1567) radius 3.05
  dimension "d821" = 3.05
  constraint coincident L0.start L1.start
  constraint coincident L0.start A0
  measures "d821" distance of L0.start L2.end
sweep "Sweep6'''''''''" cut profiles "Sketch95" along 1 edges at (-410, -77.5789, 44.7902) section 1 sketch seen with x (0, 0.5, 0.866025) y (0, 0.866025, -0.5) z (-1, 0, 0) at (347.2001, -884.7986, 455.4131) on bodies 30 bodies 30 in component "Component'''"
ref_plane "WorkPlane94" through (57, 904.3842, 347.2001) normal (-1, 0, 0) x (0, 0, -1)
sketch "Sketch96" plane through (57, 904.3842, 347.2001) normal (-1, 0, 0) x (0, 0, -1)
  line L0 (0, -84.3842) -> (0, 0) construction
  line L1 (0, 0) -> (18, 0) construction
  line L2 (0, 0) -> (2.1567, -2.1567) construction
  circle A0 centre (2.1567, -2.1567) radius 3.05
  dimension "d829" = 3.05
  constraint coincident L0.end L1.start
  constraint coincident L0.end A0
  measures "d829" distance of L0.end L2.end
sweep "Sweep7'''''''''" cut profiles "Sketch96" along 1 edges at (0, -77.5789, 44.7902) section 1 sketch seen with x (0, 0.5, 0.866025) y (0, 0.866025, -0.5) z (-1, 0, 0) at (347.2001, -884.7986, 455.4131) on bodies 30 bodies 30 in component "Component'''"
ref_plane "WorkPlane95" through (39, 814.3842, 347.2001) normal (1, 0, 0) x (0, 0, 1)
sketch "Sketch97" plane through (39, 814.3842, 347.2001) normal (1, 0, 0) x (0, 0, 1)
  line L0 (0, 0) -> (0, 84.3842) construction
  line L1 (0, 0) -> (-18, 0) construction
  line L2 (0, 0) -> (-2.1567, 2.1567) construction
  circle A0 centre (-2.1567, 2.1567) radius 3.05
  dimension "d837" = 3.05
  constraint coincident L0.start L1.start
  constraint coincident L0.start A0
  measures "d837" distance of L0.start L2.end
sweep "Sweep8'''''''''" cut profiles "Sketch97" along 1 edges at (0, -155.5211, 89.7902) section 1 sketch seen with x (0, 0.5, 0.866025) y (0, 0.866025, -0.5) z (-1, 0, 0) at (347.2001, -884.7986, 455.4131) on bodies 30 bodies 30 in component "Component'''"
ref_plane "WorkPlane96" through (57, 814.3842, 291.2001) normal (-1, 0, 0) x (0, 0, 1)
sketch "Sketch98" plane through (57, 814.3842, 291.2001) normal (-1, 0, 0) x (0, 0, 1)
  line L0 (0, 0) -> (0, -84.3842) construction
  line L1 (0, 0) -> (18, 0) construction
  line L2 (0, 0) -> (2.1567, -2.1567) construction
  circle A0 centre (2.1567, -2.1567) radius 3.05
  dimension "d845" = 3.05
  constraint coincident L0.start L1.start
  constraint coincident L0.start A0
  measures "d845" distance of L0.start L2.end
sweep "Sweep5''''''''''" cut profiles "Sketch98" along 1 edges at (-410, 77.5789, 44.7902) section 1 sketch seen with x (0, -0.5, 0.866025) y (0, 0.866025, 0.5) z (-1, 0, 0) at (-118.7999, -603.6986, -403.9712) on bodies 29 bodies 29 in component "Component''"
ref_plane "WorkPlane97" through (39, 904.3842, 291.2001) normal (1, 0, 0) x (0, 0, -1)
sketch "Sketch99" plane through (39, 904.3842, 291.2001) normal (1, 0, 0) x (0, 0, -1)
  line L0 (0, 0) -> (0, 84.3842) construction
  line L1 (0, 0) -> (-18, 0) construction
  line L2 (0, 0) -> (-2.1567, 2.1567) construction
  circle A0 centre (-2.1567, 2.1567) radius 3.05
  dimension "d853" = 3.05
  constraint coincident L0.start L1.start
  constraint coincident L0.start A0
  measures "d853" distance of L0.start L2.end
sweep "Sweep6''''''''''" cut profiles "Sketch99" along 1 edges at (-410, 155.5211, 89.7902) section 1 sketch seen with x (0, -0.5, 0.866025) y (0, 0.866025, 0.5) z (-1, 0, 0) at (-118.7999, -603.6986, -403.9712) on bodies 29 bodies 29 in component "Component''"
ref_plane "WorkPlane98" through (57, 904.3842, -118.7999) normal (-1, 0, 0) x (0, 0, 1)
sketch "Sketch100" plane through (57, 904.3842, -118.7999) normal (-1, 0, 0) x (0, 0, 1)
  line L0 (0, 0) -> (0, 84.3842) construction
  line L1 (0, 0) -> (-18, 0) construction
  line L2 (0, 0) -> (-2.1567, 2.1567) construction
  circle A0 centre (-2.1567, 2.1567) radius 3.05
  dimension "d861" = 3.05
  constraint coincident L0.start L1.start
  constraint coincident L0.start A0
  measures "d861" distance of L0.start L2.end
sweep "Sweep7''''''''''" cut profiles "Sketch100" along 1 edges at (0, 155.5211, 89.7902) section 1 sketch seen with x (0, -0.5, 0.866025) y (0, 0.866025, 0.5) z (-1, 0, 0) at (-118.7999, -603.6986, -403.9712) on bodies 29 bodies 29 in component "Component''"
ref_plane "WorkPlane99" through (39, 814.3842, -118.7999) normal (1, 0, 0) x (0, 0, -1)